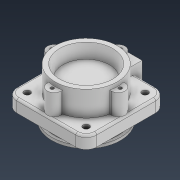
# Autodesk Inventor part: Pokrywa cylindra tyl
Saved by Autodesk Inventor 2022 (Build 260153000, 153)
## iProperties
Created: 2023-04-12
Part Number: Pokrywa cylindra tyl
Material: Generic
Document SubType Name: Modeling
Designer: wikto
Density: 1 g/cm^3
Appearance: Default
Author: wikto
Autodesk Inventor part; units mm, degrees
ref_plane "YZ Plane" through (0, 0, 0) normal (1, 0, 0) x (0, 1, 0)
ref_plane "XZ Plane" through (0, 0, 0) normal (0, 1, 0) x (-1, 0, 0)
ref_plane "XY Plane" through (0, 0, 0) normal (0, 0, 1) x (1, 0, 0)
sketch "Sketch1" plane through (0, 0, 0) normal (0, 1, 0) x (-1, 0, 0)
  line L0 (57.5, 57.5) -> (-57.5, 57.5)
  line L1 (-57.5, 57.5) -> (-57.5, -57.5)
  line L2 (-57.5, -57.5) -> (57.5, -57.5)
  line L3 (57.5, -57.5) -> (57.5, 57.5)
  line L4 (57.5, 57.5) -> (-57.5, -57.5) construction
  line L5 (-57.5, 57.5) -> (57.5, -57.5) construction
  point P0 (0, 0)
  dimension "d0" = 115
  dimension "d1" = 115
  constraints: 12 end point, 2 midpoint, 2 parallel, 1 horizontal, 1 perpendicular
  measures "d0" distance of L2.end L1.end
  measures "d1" distance of L1.end L0.end
extrude "Extrusion1" add sketch "Sketch1" along normal blind 18
sketch "Sketch2" plane through (0, 0, 0) normal (0, -1, 0) x (1, 0, 0)
  circle A0 centre (0, 0) radius 49.5
  dimension "d4" = 99
  constraints: 1 centre point, 1 coincident
  measures "d4" diameter of A0
extrude "Extrusion2" add sketch "Sketch2" along normal blind 17
sketch "Sketch3" plane through (0, 18, 0) normal (0, 1, 0) x (1, 0, 0)
  circle A0 centre (0, 0) radius 45
  dimension "d8" = 90
  constraints: 1 centre point
  measures "d8" diameter of A0
extrude "Extrusion5" add sketch "Sketch3" along normal blind 33
ref_plane "Work Plane1" through (0, 18, -45) normal (0, 0, -1) x (-1, 0, 0)
sketch "Sketch5" plane through (0, 18, -45) normal (0, 0, -1) x (-1, 0, 0)
  line L0 (12, -18) -> (-12, -18)
  line L1 (-12, -18) -> (-12, 12)
  line L2 (-12, 12) -> (12, 12)
  line L3 (12, 12) -> (12, -18)
  line L4 (12, -18) -> (-12, 12) construction
  line L5 (-12, -18) -> (12, 12) construction
  line L6 (-57.5, -18) -> (57.5, -18) projected
  point P0 (0, -18)
  point P1 (0, -3)
  point P2 (0, -18)
  point P3 (0, 12)
  point P4 (0, -18)
  dimension "d22" = 24
  dimension "d23" = 30
  constraints: 12 end point, 6 midpoint, 2 parallel, 1 horizontal, 1 perpendicular, 1 vertical alignment
  measures "d22" distance of L1.end L2.end
  measures "d23" distance of L0.end L1.end
extrude "Extrusion7" add sketch "Sketch5" along normal blind 23.5 and the other way blind 5
sketch "Sketch6" plane through (0, 18, -45) normal (0, 0, -1) x (-1, 0, 0)
  line L0 (10, 12) -> (-10, 12)
  line L1 (-10, 12) -> (-10, 30)
  line L2 (-10, 30) -> (10, 30)
  line L3 (10, 30) -> (10, 12)
  line L4 (10, 12) -> (-10, 30) construction
  line L5 (-10, 12) -> (10, 30) construction
  line L6 (12, 12) -> (-12, 12) projected
  point P0 (0, -18)
  point P1 (0, 21)
  point P2 (0, 12)
  point P3 (0, 21)
  point P4 (0, 12)
  dimension "d28" = 20
  dimension "d29" = 18
  constraints: 12 end point, 6 midpoint, 2 parallel, 1 horizontal, 1 perpendicular, 1 vertical alignment
  measures "d28" distance between parallel lines of L3 L1
  measures "d29" distance between parallel lines of L0 L2
extrude "Extrusion8" add sketch "Sketch6" along normal blind 11 and the other way blind 3
ref_plane "Work Plane2" through (0, -13, 0) normal (0, -1, 0) x (1, 0, 0)
sketch "Sketch9" plane through (0, -13, 0) normal (0, -1, 0) x (1, 0, 0)
  circle A0 centre (0, 0) radius 45.5
  circle A1 centre (0, 0) radius 49.5 projected
  dimension "d41" = 4
  constraints: 1 centre point, 1 coincident
  measures "d41" radial gap between concentric circles of A1 A0
extrude "Extrusion11" cut sketch "Sketch9" against normal blind 6
fillet "Fillet1" radius 15 4 edges at (-57.5, 9, -57.5) (57.5, 9, -57.5) (57.5, 9, 57.5) (-57.5, 9, 57.5)
full round fillet "Full Round Fillet1" first side at (-10, 36, -47.9165) centre faces at (3.3333, 36, -56) second side at (10, 36, -47.9165)
fillet "Fillet2" radius 3 9 edges at (-53.1066, 18, 53.1066) (0, 18, 57.5) (53.1066, 18, 53.1066) (57.5, 18, 0) (53.1066, 18, -53.1066) (27.25, 18, -57.5) (-53.1066, 18, -53.1066) (-27.25, 18, -57.5) (-57.5, 18, 0)
pattern_circular "Circular Pattern2" count 4 over 360 about axis through (0, -10, 0) along (0, 1, 0) of "Full Round Fillet1", "Extrusion8"
sketch "Sketch10" plane through (-46, 30, 10) normal (0, -1, 0) x (1, 0, 0)
  arc A0 (2.1252, 0) -> (2.1252, -20) centre (46, -10) ccw projected
  line L0 (2.1252, 0) -> (0, 0) projected
  arc A1 (0, 0) -> (0, -20) centre (0, -10) ccw projected
  line L1 (2.1252, -20) -> (0, -20) projected
  arc A2 (56, 33.8748) -> (36, 33.8748) centre (46, -10) ccw projected
  line L2 (56, 33.8748) -> (56, 36) projected
  arc A3 (56, 36) -> (36, 36) centre (46, 36) ccw projected
  line L3 (36, 33.8748) -> (36, 36) projected
  arc A4 (89.8748, -20) -> (89.8748, 0) centre (46, -10) ccw projected
  line L4 (89.8748, -20) -> (92, -20) projected
  arc A5 (92, -20) -> (92, 0) centre (92, -10) ccw projected
  line L5 (89.8748, 0) -> (92, 0) projected
  point P0 (46, -10)
extrude "Extrusion12" add sketch "Sketch10" along normal blind 20
sketch "Sketch11" plane through (0, 18, 0) normal (0, 1, 0) x (1, 0, 0)
  arc A0 (-42.5, 54.5) -> (-54.5, 42.5) centre (-42.5, 42.5) ccw projected
  arc A1 (-54.5, -42.5) -> (-42.5, -54.5) centre (-42.5, -42.5) ccw projected
  arc A2 (42.5, -54.5) -> (54.5, -42.5) centre (42.5, -42.5) ccw projected
  point P0 (0, 0)
  point P1 (42.5, 42.5)
  constraints: 3 coincident, 2 horizontal alignment, 2 vertical alignment
hole "Hole1" at (-42.5, 18, -42.5) at (42.5, 18, -42.5) at (42.5, 18, 42.5) at (-42.5, 18, 42.5) direction (0, -1, 0) diameter 9 end through all
sketch "Sketch13" plane through (0, 18, -68.5) normal (0, 0, -1) x (-1, 0, 0)
  line L0 (12, 12) -> (-12, 12) projected
  line L1 (-12, 12) -> (-12, -18) projected
  point P0 (0, -18)
  point P1 (0, -3)
  dimension "d74" = 15
  dimension "d75" = 12
  measures "d74" distance from line of L0 point (0, -3)
  measures "d75" distance from line of L1 point (0, -3)
hole "Hole3" at (0, 15, -68.5) direction (0, 0, 1) diameter 11.835 depth 20 tip angle 118 thread size "M14x2" class "6H" standard "ISO Metric profile"
sketch "Sketch14" plane through (0, 48, 0) normal (0, 1, 0) x (1, 0, 0)
  arc A0 (-46, 10) -> (-46, -10) centre (-46, 0) ccw projected
  arc A1 (10, 46) -> (-10, 46) centre (0, 46) ccw projected
  arc A2 (46, -10) -> (46, 10) centre (46, 0) ccw projected
  arc A3 (-10, -46) -> (10, -46) centre (0, -46) ccw projected
  point P0 (0, 0)
  point P1 (0, 49)
  point P2 (49, 0)
  point P3 (0, -49)
  point P4 (-49, 0)
  dimension "d83" = 3
  dimension "d84" = 3
  dimension "d85" = 3
  dimension "d86" = 3
  constraints: 2 horizontal alignment, 2 vertical alignment
  measures "d83" distance of point (-49, 0) A0.centre
  measures "d84" distance of A1.centre point (0, 49)
  measures "d85" distance of A2.centre point (49, 0)
  measures "d86" distance of A3.centre point (0, -49)
hole "Hole4" at (0, 48, -49) at (49, 48, 0) at (0, 48, 49) at (-49, 48, 0) direction (0, -1, 0) diameter 4.917 depth 20 tip angle 118 thread size "M6x1" class "6H" standard "ISO Metric profile"
sketch "Sketch16" plane through (0, 51, 0) normal (0, 1, 0) x (1, 0, 0)
  circle A0 centre (0, 0) radius 37.5
  dimension "d104" = 75
  constraints: 1 centre point, 1 coincident
  measures "d104" diameter of A0
extrude "Extrusion14" cut sketch "Sketch16" against normal blind 15 draft -15
sketch "Sketch18" plane through (0, -17, 0) normal (0, -1, 0) x (1, 0, 0)
  point P0 (0, 0)
  point P1 (0, 0)
  constraints: 1 coincident
hole "Hole5" at (0, -17, 0) direction (0, 1, 0) diameter 26 depth 43 counterbore diameter 32 counterbore depth 40
fillet "Fillet4" radius 2 1 edges at (0, -17, 16)
chamfer "Chamfer4" distance 2 angle 45 1 edges at (0, 26, 13)
offset faces "Size1" outward 3 faces at (42.1722, 51, -3.1187)
sketch "Sketch20" plane through (0, 18, -68.5) normal (0, 0, -1) x (-1, 0, 0)
  line L0 (-12, -18) -> (12, -18) projected
  line L1 (12, -18) -> (12, 12) projected
  point P0 (0, -18)
  point P1 (0, -3)
  dimension "d119" = 15
  dimension "d120" = 12
  measures "d119" distance from line of L0 point (0, -3)
  measures "d120" distance from line of L1 point (0, -3)
hole "Hole6" at (0, 15, -68.5) direction (0, 0, 1) diameter 10 end up to face face through (0, 3, 0) facing (0, -1, 0) round with radius 16 far side no
body "Solid1"
